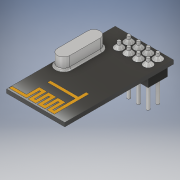
# Autodesk Inventor part: NRF24L01
Saved by Autodesk Inventor 2019.2 (Build 232265000, 265)
## iProperties
Created: 2018-12-18
Part Number: NRF24L01
Material: Acetal Resin, Black
Document SubType Name: Modeling
Designer: Petar
Density: 1.425 g/cm^3
Appearance: Chrome - Polished Black
Author: Petar
Autodesk Inventor part; units mm, degrees
ref_plane "YZ Plane" through (0, 0, 0) normal (1, 0, 0) x (0, 1, 0)
ref_plane "XZ Plane" through (0, 0, 0) normal (0, 1, 0) x (-1, 0, 0)
ref_plane "XY Plane" through (0, 0, 0) normal (0, 0, 1) x (1, 0, 0)
sketch "Sketch1" plane through (0, 0, 0) normal (0, 1, 0) x (-1, 0, 0)
  line L0 (7.5, 14) -> (-7.5, 14)
  line L1 (-7.5, 14) -> (-7.5, -14)
  line L2 (-7.5, -14) -> (7.5, -14)
  line L3 (7.5, -14) -> (7.5, 14)
  line L4 (0, 14) -> (0, -14) construction
  line L5 (7.5, 0) -> (-7.5, 0) construction
  line L6 (5.4, 3) -> (5.4, -8) construction
  line L7 (3.8, 1.4) -> (3.8, -6.4)
  line L8 (7, -6.4) -> (7, 1.4)
  arc A0 (7, 1.4) -> (3.8, 1.4) centre (5.4, 1.4) ccw
  arc A1 (3.8, -6.4) -> (7, -6.4) centre (5.4, -6.4) ccw
  line L9 (3.5, -13.5) -> (-6.5, -13.5)
  line L10 (-6.5, -13.5) -> (-6.5, -8.5)
  line L11 (-6.5, -8.5) -> (3.5, -8.5)
  line L12 (3.5, -8.5) -> (3.5, -13.5)
  line L13 (3.5, -11) -> (-6.5, -11) construction
  circle A2 centre (2.25, -12.25) radius 1.25
  circle A3 centre (2.25, -12.25) radius 0.4
  circle A4 centre (2.25, -9.75) radius 1.25
  circle A5 centre (2.25, -9.75) radius 0.4
  circle A6 centre (-0.25, -12.25) radius 1.25
  circle A7 centre (-0.25, -12.25) radius 0.4
  circle A8 centre (-0.25, -9.75) radius 1.25
  circle A9 centre (-0.25, -9.75) radius 0.4
  circle A10 centre (-2.75, -12.25) radius 1.25
  circle A11 centre (-2.75, -12.25) radius 0.4
  circle A12 centre (-2.75, -9.75) radius 1.25
  circle A13 centre (-2.75, -9.75) radius 0.4
  circle A14 centre (-5.25, -12.25) radius 1.25
  circle A15 centre (-5.25, -12.25) radius 0.4
  circle A16 centre (-5.25, -9.75) radius 1.25
  circle A17 centre (-5.25, -9.75) radius 0.4
  line L14 (7.4, 13.5) -> (2.9, 13.5)
  line L15 (2.9, 13.5) -> (2.9, 12.7)
  line L16 (3.7, 12.7) -> (7.4, 12.7)
  line L17 (7.4, 12.7) -> (7.4, 13.5)
  line L18 (2.9, 13.5) -> (3.7, 13.5)
  line L19 (3.7, 12.7) -> (3.7, 9.4)
  line L20 (3.7, 9.4) -> (2.9, 9.4)
  line L21 (2.9, 10.2) -> (2.9, 13.5)
  line L22 (3.7, 9.4) -> (1.7076, 9.4)
  line L23 (1.7076, 9.4) -> (1.7076, 10.2)
  line L24 (2.5, 10.2) -> (2.9, 10.2)
  line L25 (3.7, 10.2) -> (3.7, 9.4)
  line L26 (1.7076, 9.4) -> (2.5, 9.4)
  line L27 (2.5, 10.2) -> (2.5, 13.5)
  line L28 (2.5, 13.5) -> (1.7, 13.5)
  line L29 (1.7076, 12.7) -> (1.7076, 9.4)
  line L30 (2.5, 13.5) -> (0.5, 13.5)
  line L31 (0.5, 13.5) -> (0.5, 12.7)
  line L32 (1.3076, 12.7) -> (1.7076, 12.7)
  line L33 (2.5, 12.7) -> (2.5, 13.5)
  line L34 (0.5, 13.5) -> (1.3, 13.5)
  line L35 (1.3076, 12.7) -> (1.3076, 9.4)
  line L36 (1.3076, 9.4) -> (0.5, 9.4)
  line L37 (0.5, 10.2) -> (0.5, 13.5)
  line L38 (1.3076, 9.4) -> (-0.7, 9.4)
  line L39 (-0.7, 9.4) -> (-0.7, 10.2)
  line L40 (0.1, 10.2) -> (0.5, 10.2)
  line L41 (1.3076, 10.2) -> (1.3076, 9.4)
  line L42 (-0.7, 9.4) -> (0.1, 9.4)
  line L43 (0.1, 10.2) -> (0.1, 13.5)
  line L44 (0.1, 13.5) -> (-0.7, 13.5)
  line L45 (-0.7, 12.7) -> (-0.7, 9.4)
  line L46 (0.1, 13.5) -> (-1.9, 13.5)
  line L47 (-1.9, 13.5) -> (-1.9, 12.7)
  line L48 (0.1, 12.7) -> (0.1, 13.5)
  line L49 (-1.9, 13.5) -> (-1.1, 13.5)
  line L50 (-1.1, 12.7) -> (-1.1, 9.4)
  line L51 (-1.1, 9.4) -> (-1.9, 9.4)
  line L52 (-1.9, 10.2) -> (-1.9, 13.5)
  line L53 (-1.1, 9.4) -> (-3.1, 9.4)
  line L54 (-3.1, 9.4) -> (-3.1, 10.2)
  line L55 (-2.3, 10.2) -> (-1.9, 10.2)
  line L56 (-1.1, 10.2) -> (-1.1, 9.4)
  line L57 (-3.1, 9.4) -> (-2.3, 9.4)
  line L58 (-2.3, 10.2) -> (-2.3, 13.5)
  line L59 (-2.3, 13.5) -> (-3.1, 13.5)
  line L60 (-3.1, 12.7) -> (-3.1, 9.4)
  line L61 (-2.3, 13.5) -> (-4.3, 13.5)
  line L62 (-4.3, 13.5) -> (-4.3, 12.7)
  line L63 (-3.5, 12.7) -> (-3.1, 12.7)
  line L64 (-2.3, 12.7) -> (-2.3, 13.5)
  line L65 (-4.3, 13.5) -> (-3.5, 13.5)
  line L66 (-3.5, 4.5) -> (-4.3, 4.5)
  line L67 (-4.3, 4.5) -> (-4.3, 13.5)
  line L68 (-3.5, 6.5) -> (3.7, 6.5)
  line L69 (3.7, 6.5) -> (3.7, 7.3)
  line L70 (3.7, 7.3) -> (-3.5, 7.3)
  line L71 (-4.3, 7.3) -> (-4.3, 6.5)
  line L72 (-1.1, 12.7) -> (-0.7, 12.7)
  line L73 (-3.5, 12.7) -> (-3.5, 7.3)
  line L74 (-3.5, 6.5) -> (-3.5, 4.5)
  circle A18 centre (5.4, 0) radius 0.4
  line L75 (7, -2.5) -> (3.8, -2.5) construction
  circle A19 centre (5.4, -5) radius 0.4
  point P0 (0, 0)
  point P1 (0, 0)
  point P2 (5.4, -2.5)
  dimension "d0" = 28
  dimension "d1" = 15
  dimension "d2" = 11
  dimension "d3" = 3.2
  dimension "d4" = 0.5
  dimension "d5" = 6
  dimension "d6" = 10
  dimension "d7" = 5
  dimension "d8" = 4
  dimension "d9" = 0.5
  dimension "d10" = 2.5
  dimension "d11" = 0.8
  dimension "d14" = 2.5
  dimension "d17" = 2.5
  dimension "d22" = 0.1
  dimension "d23" = 0.5
  dimension "d51" = 4.1
  dimension "d52" = 0.8
  dimension "d53" = 0.8
  dimension "d54" = 0.8
  dimension "d57" = 0.8
  constraints: 154 end point, 36 parallel, 20 centre point, 19 perpendicular, 18 horizontal, 10 midpoint, 9 coincident, 8 collinear, 6 point on circle, 6 point on line, 6 tangent, 2 vertical, 1 symmetric about line, 29 other
  measures "d0" distance of L1.end L0.end
  measures "d1" distance between parallel lines of L1 L3
  measures "d2" distance of L6.start L6.end
  measures "d3" diameter of A1
  measures "d4" distance between parallel lines of L3 L8
  measures "d5" distance from line of L2 L6.end
  measures "d6" distance of L10.end L11.end
  measures "d7" distance of L9.end L10.end
  measures "d8" distance between parallel lines of L12 L3
  measures "d9" distance between parallel lines of L2 L9
  measures "d10" diameter of A2
  measures "d11" diameter of A3
  measures "d14" distance of A2.centre A4.centre
  measures "d17" distance of A2.centre A6.centre
  measures "d22" distance between parallel lines of L3 L17
  measures "d23" distance between parallel lines of L0 L14
  measures "d51" distance between parallel lines of L14 L22
  measures "d52" distance between parallel lines of L16 L14
  measures "d53" distance between parallel lines of L68 L70
  measures "d54" distance between parallel lines of L67 L74
  measures "d57" diameter of A18
extrude "Extrusion1" add sketch "Sketch1" against normal blind 1 contours L3 L2 L1 L0 | A0 L8 A1 L7 | L9 A2 L12 | L9 A6 A2 | A2 | A2 A4 L12 | L9 A10 A6 | A6 | A6 A8 A4 A2 | A4 L11 L12 | A4 | L9 A14 A10 | A10 | A10 A12 A8 A6 | A8 | A4 A8 L11 | L9 L10 A14 | A14 | A14 A16 A12 A10 | A12 | A12 L11 A8 | L10 A16 A14 | A16 | A16 L11 A12 | L10 L11 A16 | A3 | A5 | A7 | A9 | A11 | A13 | A15 | A17 | L17 L16 L19 L20 L22 L23 L29 L32 L35 L36 L38 L39 L45 L72 L50 L51 L53 L54 L60 L63 L73 L70 L69 L68 L74 L66 L67 L62 L61 L59 L58 L55 L52 L47 L46 L44 L43 L40 L37 L31 L30 L28 L27 L24 L21 L15 L14 | A18 | A19
extrude "Extrusion2" add sketch "Sketch1" along normal blind 3 contours A0 L8 A1 L7 | A18 | A19
fillet "Fillet1" radius 0.5 4 edges at (-5.4, 0, 3) (-7, 0, -2.5) (-5.4, 0, -8) (-3.8, 0, -2.5)
extrude "Extrusion5" add sketch "Sketch1" against normal blind 2.5 contours A18 | A19
chamfer "Chamfer2" distance 0.75 angle 45 2 edges at (-5, -1, -5) (-5, -1, 0)
extrude "Extrusion3" add sketch "Sketch1" along normal blind 1.5 and the other way blind 10 contours A3 | A5 | A7 | A9 | A11 | A13 | A15 | A17
chamfer "Chamfer1" distance 0.75 angle 45 8 edges at (0.65, 0, -9.75) (-1.85, 0, -9.75) (-1.85, 0, -12.25) (0.65, 0, -12.25) (3.15, 0, -12.25) (3.15, 0, -9.75) (5.65, 0, -9.75) (5.65, 0, -12.25)
extrude "Extrusion4" add sketch "Sketch1" against normal blind 4 contours L9 A2 L12 | L9 A6 A2 | A2 | A2 A4 L12 | L9 A10 A6 | A6 | A6 A8 A4 A2 | A4 L11 L12 | A4 | L9 A14 A10 | A10 | A10 A12 A8 A6 | A8 | A4 A8 L11 | L9 L10 A14 | A14 | A14 A16 A12 A10 | A12 | A12 L11 A8 | L10 A16 A14 | A16 | A16 L11 A12 | L10 L11 A16 | A3 | A5 | A7 | A9 | A11 | A13 | A15 | A17
emboss "Emboss2" sketch "Sketch1" operation add depth 0.01 direction (0, -1, 0) contours L9 A2 L12 | L9 A6 A2 | A2 A4 L12 | L9 A10 A6 | A6 A8 A4 A2 | A4 L11 L12 | L9 A14 A10 | A10 A12 A8 A6 | A4 A8 L11 | L9 L10 A14 | A14 A16 A12 A10 | A12 L11 A8 | L10 A16 A14 | A16 L11 A12 | L10 L11 A16
emboss "Emboss1" sketch "Sketch1" operation add depth 0.01 direction (0, -1, 0) contours L17 L16 L19 L20 L22 L23 L29 L32 L35 L36 L38 L39 L45 L72 L50 L51 L53 L54 L60 L63 L73 L70 L69 L68 L74 L66 L67 L62 L61 L59 L58 L55 L52 L47 L46 L44 L43 L40 L37 L31 L30 L28 L27 L24 L21 L15 L14
body "Solid1" dims "d53" = 0.8
